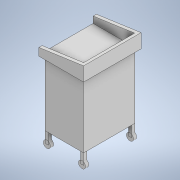
# Autodesk Inventor part: 傳統主席台
Saved by Autodesk Inventor 2021 (Build 250183000, 183)
## iProperties
Created: 2023-02-20
Part Number: 傳統主席台
Material: 一般
Document SubType Name: Modeling
Designer: brian
Density: 1 g/cm^3
Appearance: 預設
Author: brian
Autodesk Inventor part; units mm, degrees
ref_plane "YZ Plane" through (0, 0, 0) normal (1, 0, 0) x (0, 1, 0)
sketch "草圖1" plane through (0, 0, 0) normal (0, 1, 0) x (-1, 0, 0)
  line L0 (300, 400) -> (-300, 400)
  line L1 (-300, 400) -> (-300, -400)
  line L2 (-300, -400) -> (300, -400)
  line L3 (300, -400) -> (300, 400)
  line L4 (300, 400) -> (-300, -400) construction
  line L5 (-300, 400) -> (300, -400) construction
  point P0 (0, 0)
  dimension "d0" = 600
  dimension "d1" = 800
  constraints: 12 end point, 2 midpoint, 2 parallel, 1 horizontal, 1 perpendicular
  measures "d0" distance of L2.end L1.end
  measures "d1" distance of L1.end L0.end
extrude "擠出1" add sketch "草圖1" along normal blind 1200
sketch "草圖2" plane through (0, 1200, 0) normal (0, 1, 0) x (1, 0, 0)
  line L0 (-300, -400) -> (300, -400) projected
  line L1 (300, -400) -> (300, 400) projected
  line L2 (300, 400) -> (-300, 400) projected
  line L3 (-300, 400) -> (-300, -400) projected
  line L4 (350, 450) -> (350, -450)
  line L5 (350, -450) -> (-350, -450)
  line L6 (-350, -450) -> (-350, 450)
  line L7 (-350, 450) -> (350, 450)
  point P0 (0, 0)
  dimension "d4" = 50
  constraints: 8 end point, 3 other
  measures "d4" distance between parallel lines of L1 L4
extrude "擠出2" add sketch "草圖2" along normal blind 200
ref_plane "工作平面1" through (350, 1400, -450) normal (0.1414214, -0.9899495, 0) x (0, 0, 1)
split "分割1" plane through (350, 1400, -450) removes the side toward (-0.1414214, 0.9899495, 0)
sketch "草圖3" plane through (-300, 1200, 400) normal (1, 0, 0) x (0, 0, -1)
  line L0 (800, 107.1429) -> (0, 107.1429) projected
  line L1 (0, 0) -> (0, 107.1429) projected
  line L2 (800, 0) -> (0, 0) projected
  line L3 (800, 0) -> (800, 107.1429) projected
  point P0 (400, -1200)
extrude "擠出3" cut sketch "草圖3" against normal through all
sketch "草圖4" plane through (0, 1200, 0) normal (0, -1, 0) x (1, 0, 0)
  line L0 (-350, 400) -> (-300, 400) projected
  line L1 (-300, 400) -> (300, 400) projected
  line L2 (300, 400) -> (300, -400) projected
  line L3 (300, -400) -> (-300, -400) projected
  line L4 (-300, -400) -> (-350, -400) projected
  line L5 (-350, -450) -> (-350, -400) projected
  line L6 (350, -450) -> (-350, -450) projected
  line L7 (350, 450) -> (350, -450) projected
  line L8 (-350, 450) -> (350, 450) projected
  line L9 (-350, 400) -> (-350, 450) projected
  line L10 (-350, -450) -> (-350, -400) projected
  line L11 (-350, 400) -> (-300, 400) projected
  line L12 (-350, -400) -> (-350, 400)
  point P0 (0, 0)
  constraints: 2 end point, 1 vertical
extrude "擠出4" add sketch "草圖4" along normal blind 20
sketch "草圖5" plane through (0, 0, 0) normal (0, -1, 0) x (1, 0, 0)
  line L0 (-300, 400) -> (300, 400) projected
  line L1 (-300, -400) -> (-300, 400) projected
  line L2 (300, -400) -> (-300, -400) projected
  line L3 (300, 400) -> (300, -400) projected
  line L4 (-300, -400) -> (-300, 400) projected
  line L5 (-300, 350) -> (300, 350)
  line L6 (-300, -350) -> (300, -350)
  line L7 (300, 400) -> (300, -400) projected
  line L8 (-300, 400) -> (300, 400) projected
  line L9 (-250, 400) -> (-250, -400)
  line L10 (300, -400) -> (-300, -400) projected
  line L11 (250, 400) -> (250, -400)
  point P0 (0, 0)
  point P1 (-250, -350)
  point P2 (250, -350)
  point P3 (250, 350)
  point P4 (-250, 350)
  dimension "d11" = 50
  dimension "d12" = 50
  dimension "d13" = 50
  dimension "d14" = 50
  constraints: 8 end point, 8 point on line, 3 perpendicular, 1 horizontal
  measures "d11" distance between parallel lines of L0 L5
  measures "d12" distance between parallel lines of L1 L9
  measures "d13" distance between parallel lines of L3 L11
  measures "d14" distance between parallel lines of L2 L6
extrude "擠出5" cut sketch "草圖5" against normal blind 170 contours L0 L11 L5 L9 | L5 L9 L6 L1 | L5 L11 L6 L9 | L5 L3 L6 L11 | L6 L11 L2 L9
sketch "草圖6" plane through (-300, 1180, 400) normal (0, 0, 1) x (1, 0, 0)
  line L0 (50, -1180) -> (0, -1180) projected
  circle A0 centre (25, -1180) radius 54.964
  point P0 (300, -1180)
  constraints: 1 centre point, 1 midpoint
extrude "擠出6" add sketch "草圖6" against normal up to surface (50 mm away) separate body
mirror "鏡射1" about plane through (0, 0, 0) normal (1, 0, 0) bodies 2
mirror "鏡射2" about plane through (0, 0, 0) normal (0, 0, 1) bodies 2
ref_plane "工作平面2" through (0, 170, 0) normal (0, -1, 0) x (1, 0, 0)
split body "分割2" result two bodies by plane through (0, 170, 0) normal (0, -1, 0) bodies 1 first body at (-283.3333, 56.6667, -350.5) (-299.5, 113.3333, 366.6667) (283.3333, 56.6667, 350.5) (299.5, 113.3333, -366.6667)
equation "\"d12\" = d11"
equation "\"d13\" = d12"
equation "\"d14\" = d12"
